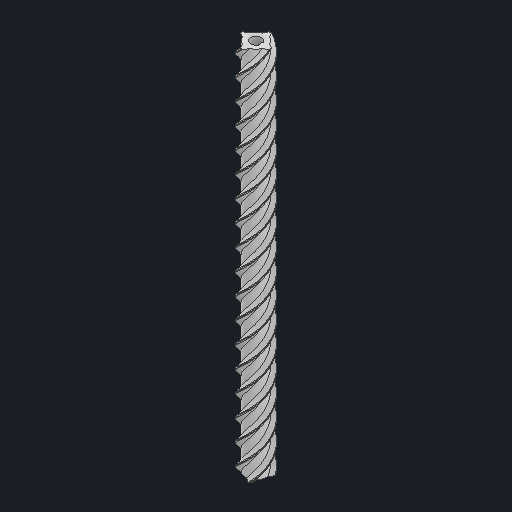
# Autodesk Inventor part: lead_screw
Saved by Autodesk Inventor 2025 (Build 290162010, 162A)
## iProperties
Created: 2024-06-23
Part Number: lead_screw
Material: Generic
Document SubType Name: Modeling
Designer: mihir
Density: 1 g/cm^3
Appearance: Default
Author: mihir
Autodesk Inventor part; units mm, degrees
ref_plane "YZ Plane" through (0, 0, 0) normal (1, 0, 0) x (0, 1, 0)
ref_plane "XZ Plane" through (0, 0, 0) normal (0, 1, 0) x (-1, 0, 0)
ref_plane "XY Plane" through (0, 0, 0) normal (0, 0, 1) x (1, 0, 0)
sketch "Sketch1" plane through (0, 0, 0) normal (0, 1, 0) x (-1, 0, 0)
  circle A0 centre (0, 0) radius 5
  dimension "d0" = 10
  constraints: 1 centre point, 1 coincident
  measures "d0" diameter of A0
extrude "Extrusion1" add sketch "Sketch1" along normal blind 177
sketch "Sketch2" plane through (0, 177, 0) normal (0, 1, 0) x (1, 0, 0)
  arc A0 (2.2517, 1.3) -> (2.2517, -1.3) centre (0, 0) ccw
  line L0 (2.2517, -1.3) -> (2.2517, 1.3)
  dimension "d3" = 2.6
  dimension "d4" = 2.6
  constraints: 2 end point, 2 point on circle, 1 centre point, 1 coincident, 1 vertical
  measures "d3" radius of A0
  measures "d4" distance of L0.start L0.end
extrude "Extrusion2" cut sketch "Sketch2" against normal up to surface (177 mm away)
sketch "Sketch3" plane through (0, 177, 0) normal (0, 1, 0) x (1, 0, 0)
  circle A0 centre (0, 0) radius 5 projected
  circle A1 centre (0, 0) radius 6.875 construction
  line L0 (-5, 0) -> (-6.8568, 0)
  line L1 (-6.8568, 0) -> (-6.8568, 0.5)
  line L2 (-6.8568, 0.5) -> (-4.6815, 1.7559)
  circle A2 centre (0, 0) radius 5 projected
  line L3 (-4.6815, 1.7559) -> (-5, 0)
  line L4 (-5, 0) -> (0, 0) construction
  line L5 (-6.8568, 0) -> (-6.8568, -0.5)
  line L6 (-6.8568, -0.5) -> (-4.6815, -1.7559)
  line L7 (-4.6815, -1.7559) -> (-5, 0)
  dimension "d21" = 13.75
  dimension "d22" = 120
  dimension "d23" = 0.5
  constraints: 16 end point, 2 horizontal, 2 symmetric about line, 1 coincident, 1 horizontal alignment, 1 perpendicular, 1 point on circle, 4 other
  measures "d23" distance of L0.end L1.end
coil "Coil1" sketch "Sketch3" operation add axis through (0, 177, 0) along (0, -1, 0) pitch 40 turns 4.425 hand right contours A0 L0 L1 L2 | L6 L5 L0 A0 | A0 L7
pattern_circular "Circular Pattern1" count 4 over 360 about axis through (0, 177, 0) along (0, 1, 0) of "Coil1"
equation "\"d0\" = lead_screw_diameter"
equation "\"d1\" = lead_screw_length"
equation "\"d3\" = motor_shaft_radius"
equation "\"d4\" = motor_shaft_radius"
equation "\"d5\" = lead_screw_length"
equation "\"d21\" = screw_outer_diameter"
equation "\"d22\" = screw_profile_angle"
equation "\"d23\" = 0.5 * screw_profile_width"
equation "\"d10\" = screw_pitch"
equation "\"lead_screw_diameter\" = 10"
equation "\"lead_screw_length\" = 177"
equation "\"motor_shaft_radius\" = 2.6"
equation "\"screw_pitch\" = 40"
equation "\"screw_outer_diameter\" = 13.75"
equation "\"screw_profile_angle\" = 120deg"
equation "\"screw_profile_width\" = 1"
body "Solid1"
